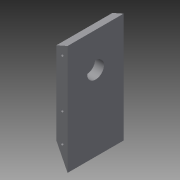
# Autodesk Inventor part: bocnice_delsi
Saved by Autodesk Inventor 2015 (Build 190159000, 159)
## iProperties
Created: 2015-01-01
Part Number: bocnice_delsi
Material: Generic
Document SubType Name: Modeling
Designer: Turboslimak
Density: 1 g/cm^3
Appearance: Default
Author: Turboslimak
Autodesk Inventor part; units mm, degrees
ref_plane "YZ Plane" through (0, 0, 0) normal (1, 0, 0) x (0, 1, 0)
ref_plane "XZ Plane" through (0, 0, 0) normal (0, 1, 0) x (-1, 0, 0)
ref_plane "XY Plane" through (0, 0, 0) normal (0, 0, 1) x (1, 0, 0)
sketch "Sketch1" plane through (0, 0, 0) normal (0, 1, 0) x (-1, 0, 0)
  line L0 (5, -36.75) -> (5, 36.75)
  line L1 (-5, 36.75) -> (-5, -36.75)
  line L2 (-5, 36.75) -> (-5, 41.1944)
  line L3 (5, 36.75) -> (-5, 41.1944)
  line L4 (-5, -36.75) -> (-5, -56.75)
  line L5 (-5, -56.75) -> (5, -36.75)
  line L6 (5, 11.25) -> (5, -36.75)
  line L7 (5, -31.75) -> (5, -36.75)
  line L8 (5, 31.75) -> (5, 36.75)
  circle A0 centre (0, 31.75) radius 1.25
  circle A1 centre (0, -36.75) radius 1.25
  circle A2 centre (0, -11.25) radius 1.25
  point P0 (0, 0)
  dimension "d3" = 10
  dimension "d4" = 73.5
  dimension "d6" = 4.4444
  dimension "d8" = 20
  dimension "d17" = 2.5
  dimension "d26" = 2.5
  dimension "d28" = 2.5
  constraints: 18 end point, 3 centre point, 2 vertical, 1 parallel
  measures "d3" distance of L1.start L0.end
  measures "d4" distance of L0.end L0.start
  measures "d6" distance of L1.start L2.end
  measures "d8" distance of L1.end L4.end
  measures "d17" diameter of A0
  measures "d26" diameter of A1
  measures "d28" diameter of A2
ref_plane "Work Plane1" through (-5, 0, -36.75) normal (-1, 0, 0) x (0, 0, 1)
extrude "Extrusion3" add sketch "Sketch1" along normal blind 50
sketch "Sketch3" plane through (-5, 0, -36.75) normal (-1, 0, 0) x (0, 0, 1)
  line L0 (73.5, 50) -> (47, 50)
  line L1 (47, 50) -> (47, 25)
  line L2 (47, 25) -> (73.5, 25)
  line L3 (73.5, 25) -> (73.5, 50)
  circle A0 centre (47, 25) radius 7.5
  circle A1 centre (47, 25) radius 4
  point P0 (36.75, 0)
  dimension "d37" = 26.5
  dimension "d38" = 25
  dimension "d39" = 15
  dimension "d42" = 8
  constraints: 8 end point, 2 centre point, 2 coincident, 2 parallel, 1 horizontal, 1 perpendicular
  measures "d37" distance of L2.end L1.end
  measures "d38" distance of L1.end L0.end
  measures "d39" diameter of A0
  measures "d42" diameter of A1
extrude "Extrusion6" cut sketch "Sketch3" against normal blind 10 contours A0 L2 A1 L1 | L1 A1 L2 A0 | A1 L2 L1 | L1 L2 A1
extrude "Extrusion7" add sketch "Sketch3" against normal blind 2 contours A0 L2 A1 L1 | L1 A1 L2 A0
body "Solid2"
